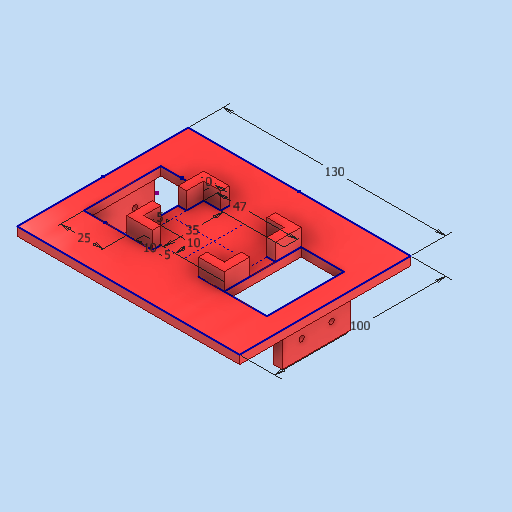
# Autodesk Inventor part: Chasis 3
Saved by Autodesk Inventor 2026.2 (Build 302298010, 298A)
## iProperties
Created: 2025-12-05
Part Number: Chasis 3
Material: Generic
Document SubType Name: Modeling
Designer: maxim
Density: 1 g/cm^3
Appearance: Light Red
Author: maxim
Autodesk Inventor part; units mm, degrees
ref_plane "YZ Plane" through (0, 0, 0) normal (1, 0, 0) x (0, 1, 0)
ref_plane "XZ Plane" through (0, 0, 0) normal (0, 1, 0) x (-1, 0, 0)
ref_plane "XY Plane" through (0, 0, 0) normal (0, 0, 1) x (1, 0, 0)
sketch "Sketch1" plane through (0, 0, 0) normal (0, 1, 0) x (-1, 0, 0)
  line L0 (0, 0) -> (-130, 0)
  line L1 (-130, 0) -> (-130, -100)
  line L2 (-130, -100) -> (0, -100)
  line L3 (0, -100) -> (0, 0)
  line L4 (-41.5, -67.5) -> (-88.5, -67.5) construction
  line L5 (-88.5, -67.5) -> (-88.5, -32.5) construction
  line L6 (-88.5, -32.5) -> (-41.5, -32.5) construction
  line L7 (-41.5, -32.5) -> (-41.5, -67.5) construction
  line L8 (-41.5, -50) -> (-88.5, -50) construction
  line L9 (-65, -67.5) -> (-65, -32.5) construction
  line L10 (-41.5, -32.5) -> (-41.5, -42.5)
  line L11 (-36.5, -42.5) -> (-41.5, -42.5)
  line L12 (-36.5, -42.5) -> (-36.5, -27.5)
  line L13 (-36.5, -27.5) -> (-51.5, -27.5)
  line L14 (-51.5, -27.5) -> (-51.5, -32.5)
  line L15 (-51.5, -32.5) -> (-41.5, -32.5)
  line L16 (-93.5, -42.5) -> (-88.5, -42.5)
  line L17 (-93.5, -42.5) -> (-93.5, -27.5)
  line L18 (-93.5, -27.5) -> (-78.5, -27.5)
  line L19 (-78.5, -27.5) -> (-78.5, -32.5)
  line L20 (-78.5, -32.5) -> (-88.5, -32.5)
  line L21 (-88.5, -42.5) -> (-88.5, -32.5)
  line L22 (-36.5, -57.5) -> (-41.5, -57.5)
  line L23 (-36.5, -57.5) -> (-36.5, -72.5)
  line L24 (-36.5, -72.5) -> (-51.5, -72.5)
  line L25 (-51.5, -72.5) -> (-51.5, -67.5)
  line L26 (-93.5, -57.5) -> (-88.5, -57.5)
  line L27 (-93.5, -57.5) -> (-93.5, -72.5)
  line L28 (-93.5, -72.5) -> (-78.5, -72.5)
  line L29 (-78.5, -72.5) -> (-78.5, -67.5)
  line L30 (-41.5, -57.5) -> (-41.5, -67.5)
  line L31 (-51.5, -67.5) -> (-41.5, -67.5)
  line L32 (-78.5, -67.5) -> (-88.5, -67.5)
  line L33 (-88.5, -57.5) -> (-88.5, -67.5)
  line L34 (-11.5, -72.5) -> (-36.5, -72.5)
  line L35 (-36.5, -72.5) -> (-36.5, -27.5)
  line L36 (-36.5, -27.5) -> (-11.5, -27.5)
  line L37 (-11.5, -27.5) -> (-11.5, -72.5)
  line L38 (-118.5, -72.5) -> (-93.5, -72.5)
  line L39 (-93.5, -72.5) -> (-93.5, -27.5)
  line L40 (-93.5, -27.5) -> (-118.5, -27.5)
  line L41 (-118.5, -27.5) -> (-118.5, -72.5)
  point P0 (0, -50)
  point P1 (-65, -100)
  point P2 (-24, -72.5)
  point P3 (-24, -57.5)
  point P4 (-24, -27.5)
  dimension "d0" = 130
  dimension "d1" = 100
  dimension "d4" = 47
  dimension "d5" = 35
  dimension "d6" = 5
  dimension "d7" = 5
  dimension "d8" = 10
  dimension "d9" = 10
  dimension "d26" = 25
  dimension "d27" = 0
  constraints: 84 end point, 19 symmetric about line, 8 midpoint, 7 perpendicular, 6 parallel, 4 collinear, 4 horizontal, 3 horizontal alignment, 2 point on line, 2 vertical, 2 vertical alignment
  measures "d0" distance of L2.end L1.end
  measures "d1" distance of L1.end L0.end
  measures "d4" distance of L4.start L4.end
  measures "d5" distance of L4.end L5.end
  measures "d6" distance of L13.end L14.end
  measures "d7" distance of L11.start L10.end
  measures "d8" distance from line of L11 L6.end
  measures "d9" distance of L14.end L6.end
  measures "d26" distance of L35.end L36.end
  measures "d27" distance between parallel lines of L23 L35
extrude "Extrusion1" add sketch "Sketch1" against normal blind 5 contours L3 L2 L1 L0 | L15 L14 L13 L12 L11 L10 | L23 L24 L25 L31 L30 L22 | L17 L18 L19 L20 L21 L16 | L26 L33 L32 L29 L28 L27
extrude "Extrusion2" add sketch "Sketch1" along normal blind 10 contours L15 L14 L13 L12 L11 L10 | L23 L24 L25 L31 L30 L22 | L17 L18 L19 L20 L21 L16 | L26 L33 L32 L29 L28 L27
sketch "Sketch2" plane through (0, -5, 0) normal (0, -1, 0) x (1, 0, 0)
  line L0 (120, -30) -> (125, -30)
  line L1 (125, -30) -> (125, -70)
  line L2 (125, -70) -> (120, -70)
  line L3 (120, -70) -> (120, -30)
  line L4 (130, -100) -> (130, 0) projected
  line L5 (0, 0) -> (130, 0) projected
  line L6 (65, 0) -> (65, -100) construction
  line L7 (130, -100) -> (0, -100) projected
  line L8 (10, -30) -> (5, -30)
  line L9 (5, -30) -> (5, -70)
  line L10 (5, -70) -> (10, -70)
  line L11 (10, -70) -> (10, -30)
  point P0 (125, -50)
  point P1 (130, -50)
  dimension "d12" = 5
  dimension "d13" = 40
  dimension "d14" = 5
  constraints: 18 end point, 4 midpoint, 4 symmetric about line, 2 parallel, 1 horizontal, 1 horizontal alignment, 1 perpendicular
  measures "d12" distance of L1.end L2.end
  measures "d13" distance of L0.end L1.end
  measures "d14" distance between parallel lines of L4 L1
extrude "Extrusion3" add sketch "Sketch2" along normal blind 20
sketch "Sketch3" plane through (5, -5, -70) normal (-1, 0, 0) x (0, 0, 1)
  line L0 (11.25, -10) -> (28.75, -10) construction
  line L1 (70, 0) -> (-30, 0) projected
  point P0 (70, 5)
  point P1 (20, 0)
  point P2 (20, -10)
  dimension "d17" = 17.5
  dimension "d18" = 10
  constraints: 2 coincident, 2 end point, 2 midpoint, 1 horizontal, 1 vertical alignment
  measures "d17" distance of L0.start L0.end
  measures "d18" distance between parallel lines of L1 L0
hole "Hole1" at (5, -15, -41.25) at (5, -15, -58.75) direction (1, 0, 0) diameter 3.1 end through all
body "Solid1"
